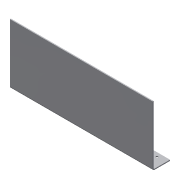
# Autodesk Inventor part: 17-0028-0024
Saved by Autodesk Inventor 2016 SP2 (Build 200236200, 236)
## iProperties
Category: IOP
Company: Universiteit van Amsterdam
Created: 2017-11-02
Part Number: 17-0028-0024
Material: Aluminum-6061-T6
Document SubType Name: Sheet Metal
Designer: Daan Giesen
Density: 2.71 g/cm^3
Sheet Metal Rule: Default_mm
Appearance: Aluminum - Flat - Version 1.1
Mass: 225.611 g
Surface Area: 873.904 cm^2
Volume: 83.2511 cm^3
Project: Digital PID Loop
Cost Center: 17-0028
User Status: Work in Progress
Authority: Reichsöllner, Lukas
Description: single bank frame
Author: Daan Giesen
Title: Digital PID Loop
Revision Number: A
Autodesk Inventor part; units mm, degrees
ref_plane "YZ Plane" through (0, 0, 0) normal (1, 0, 0) x (0, 1, 0)
ref_plane "XZ Plane" through (0, 0, 0) normal (0, 1, 0) x (-1, 0, 0)
ref_plane "XY Plane" through (0, 0, 0) normal (0, 0, 1) x (1, 0, 0)
sketch "Sketch1" plane through (0, 0, 0) normal (0, 0, 1) x (1, 0, 0)
  line L0 (0, 84) -> (0, -84) construction
  line L1 (-198.8, 0) -> (198.8, 0) construction
  line L2 (-142, -60) -> (142, -60)
  line L3 (142, -60) -> (142, 60)
  line L4 (142, 60) -> (-142, 60)
  line L5 (-142, 60) -> (-142, -60)
  line L6 (-142, -60) -> (142, 60) construction
  line L7 (142, -60) -> (-142, 60) construction
  point P0 (0, 0)
  dimension "d0" = 284
  dimension "d1" = 120
  measures "d0" distance of L3.end L4.end
  measures "d1" distance of L2.end L3.end
extrude "Plate1" add sketch "Sketch1" along normal blind 2
sketch "Sketch2" plane through (-142, -58, 2) normal (0, -1, 0) x (1, 0, 0)
  line L0 (284, 0) -> (0, 0)
  line L1 (0, 0) -> (0, -35)
  line L2 (0, -35) -> (284, -35)
  line L3 (284, -35) -> (284, 0)
  constraints: 6 end point, 1 horizontal, 1 perpendicular, 1 vertical
edge flange "Flange1" height 35 angle 90 thickness 2 bend radius 2 thickness toward (0, -1, 0) relief tear relief width 2 relief depth 1 edges at (0, -60, 0) wall of the first edge with corners at (142, -58, 2) (-142, -58, 2) (-142, -58, -33) (142, -58, -33)
bend "Bend1"
corner "Corner1"
sketch "Sketch5" plane through (0, 0, 2) normal (0, 0, 1) x (1, 0, 0)
  circle A0 centre (-111.95, 42.639) radius 2 projected
  circle A1 centre (-85.95, 42.639) radius 2 projected
  circle A2 centre (-59.95, 42.639) radius 2 projected
  circle A3 centre (-33.95, 42.639) radius 2 projected
  circle A4 centre (-7.95, 42.639) radius 2 projected
  circle A5 centre (25.35, 42.639) radius 2 projected
  circle A6 centre (51.35, 42.639) radius 2 projected
  circle A7 centre (77.35, 42.639) radius 2 projected
  circle A8 centre (103.35, 42.639) radius 2 projected
  circle A9 centre (129.35, 42.639) radius 2 projected
  circle A10 centre (116.35, 42.639) radius 2 projected
  circle A11 centre (90.35, 42.639) radius 2 projected
  circle A12 centre (64.35, 42.639) radius 2 projected
  circle A13 centre (38.35, 42.639) radius 2 projected
  circle A14 centre (12.35, 42.639) radius 2 projected
  circle A15 centre (-20.95, 42.639) radius 2 projected
  circle A16 centre (-46.95, 42.639) radius 2 projected
  circle A17 centre (-72.95, 42.639) radius 2 projected
  circle A18 centre (-98.95, 42.639) radius 2 projected
  circle A19 centre (-124.95, 42.639) radius 2 projected
  circle A20 centre (12, 52) radius 2.65 projected
  circle A21 centre (52, 52) radius 2.65 projected
  circle A22 centre (92, 52) radius 2.65 projected
  circle A23 centre (132, 52) radius 2.65 projected
  circle A24 centre (112, 26) radius 2.65 projected
  circle A25 centre (72, 26) radius 2.65 projected
  circle A26 centre (32, 26) radius 2.65 projected
  circle A27 centre (-8, 26) radius 2.65 projected
  circle A28 centre (-48, 26) radius 2.65 projected
  circle A29 centre (-28, 52) radius 2.65 projected
  circle A30 centre (-68, 52) radius 2.65 projected
  circle A31 centre (-88, 52) radius 2.65 projected
  circle A32 centre (-108, 52) radius 2.65 projected
  circle A33 centre (-128, 52) radius 2.65 projected
  circle A34 centre (-118, -8) radius 2.65 projected
  circle A35 centre (-95.7, 5) radius 2.65 projected
  circle A36 centre (-69.7, 5) radius 2.65 projected
  circle A37 centre (-43.7, 5) radius 2.65 projected
  circle A38 centre (-17.7, 5) radius 2.65 projected
  circle A39 centre (2.3, 5) radius 2.65 projected
  circle A40 centre (28.3, 5) radius 2.65 projected
  circle A41 centre (54.3, 5) radius 2.65 projected
  circle A42 centre (80.3, 5) radius 2.65 projected
  circle A43 centre (106.3, 5) radius 2.65 projected
  circle A44 centre (132.3, 5) radius 2.65 projected
  circle A45 centre (136, -8) radius 2.65 projected
  circle A46 centre (110, -8) radius 2.65 projected
  circle A47 centre (84, -8) radius 2.65 projected
  circle A48 centre (58, -8) radius 2.65 projected
  circle A49 centre (32, -8) radius 2.65 projected
  circle A50 centre (6, -8) radius 2.65 projected
  circle A51 centre (-14, -8) radius 2.65 projected
  circle A52 centre (-40, -8) radius 2.65 projected
  circle A53 centre (-66, -8) radius 2.65 projected
  circle A54 centre (-92, -8) radius 2.65 projected
  circle A55 centre (-121.7, 5) radius 2.65 projected
  circle A56 centre (-128, 26) radius 2.65 projected
  circle A57 centre (-108, 26) radius 2.65 projected
  circle A58 centre (-88, 26) radius 2.65 projected
  circle A59 centre (-48, 52) radius 2.65 projected
  circle A60 centre (-68, 26) radius 2.65 projected
  circle A61 centre (-28, 26) radius 2.65 projected
  circle A62 centre (12, 26) radius 2.65 projected
  circle A63 centre (52, 26) radius 2.65 projected
  circle A64 centre (92, 26) radius 2.65 projected
  circle A65 centre (132, 26) radius 2.65 projected
  circle A66 centre (112, 52) radius 2.65 projected
  circle A67 centre (72, 52) radius 2.65 projected
  circle A68 centre (32, 52) radius 2.65 projected
  circle A69 centre (-8, 52) radius 2.65 projected
  line L0 (-142, -15) -> (142, -15) projected
  line L1 (-142, 60) -> (-142, -15) projected
  line L2 (142, 60) -> (-142, 60) construction
  line L3 (142, -15) -> (142, 60) projected
  line L4 (142, -47.8) -> (142, -19.2) projected
  arc A70 (142, -19.2) -> (139.8, -17) centre (139.8012, -19.1988) ccw projected
  line L5 (139.8, -17) -> (-139.8, -17) construction
  arc A71 (-139.8, -17) -> (-142, -19.2) centre (-139.8012, -19.1988) ccw projected
  line L6 (-142, -19.2) -> (-142, -47.8) projected
  arc A72 (-142, -47.8) -> (-139.8, -50) centre (-139.8012, -47.8012) ccw projected
  line L7 (-139.8, -50) -> (139.8, -50) projected
  arc A73 (139.8, -50) -> (142, -47.8) centre (139.8012, -47.8012) ccw projected
  circle A74 centre (138, -46) radius 1.6 projected
  circle A75 centre (123.9, -21.55) radius 0.5 projected
  circle A76 centre (84.9, -21.55) radius 0.5 projected
  circle A77 centre (93.4, -21.55) radius 0.5 projected
  circle A78 centre (138, -21) radius 1.6 projected
  circle A79 centre (132.4, -21.55) radius 0.5 projected
  circle A80 centre (106.4, -21.55) radius 0.5 projected
  circle A81 centre (119.4, -21.55) radius 0.5 projected
  circle A82 centre (110.9, -21.55) radius 0.5 projected
  circle A83 centre (45.9, -21.55) radius 0.5 projected
  circle A84 centre (54.4, -21.55) radius 0.5 projected
  circle A85 centre (1, -46) radius 1.6 projected
  circle A86 centre (28.4, -21.55) radius 0.5 projected
  circle A87 centre (1, -27) radius 1.6 projected
  circle A88 centre (71.9, -21.55) radius 0.5 projected
  circle A89 centre (80.4, -21.55) radius 0.5 projected
  circle A90 centre (-13.4, -21.55) radius 0.5 projected
  circle A91 centre (19.9, -21.55) radius 0.5 projected
  circle A92 centre (-4.9, -21.55) radius 0.5 projected
  circle A93 centre (97.9, -21.55) radius 0.5 projected
  circle A94 centre (128.15, -21.55) radius 0.5 projected
  circle A95 centre (58.9, -21.55) radius 0.5 projected
  circle A96 centre (67.4, -21.55) radius 0.5 projected
  circle A97 centre (102.15, -21.55) radius 0.5 projected
  circle A98 centre (115.15, -21.55) radius 0.5 projected
  circle A99 centre (89.15, -21.55) radius 0.5 projected
  circle A100 centre (76.15, -21.55) radius 0.5 projected
  circle A101 centre (63.15, -21.55) radius 0.5 projected
  circle A102 centre (41.4, -21.55) radius 0.5 projected
  circle A103 centre (50.15, -21.55) radius 0.5 projected
  circle A104 centre (6.9, -21.55) radius 0.5 projected
  circle A105 centre (32.9, -21.55) radius 0.5 projected
  circle A106 centre (15.4, -21.55) radius 0.5 projected
  circle A107 centre (24.15, -21.55) radius 0.5 projected
  circle A108 centre (37.15, -21.55) radius 0.5 projected
  circle A109 centre (-9.15, -21.55) radius 0.5 projected
  circle A110 centre (11.15, -21.55) radius 0.5 projected
  circle A111 centre (1, -21) radius 0.5 projected
  circle A112 centre (-52.4, -21.55) radius 0.5 projected
  circle A113 centre (-43.9, -21.55) radius 0.5 projected
  circle A114 centre (-128, -46) radius 1.6 projected
  circle A115 centre (-69.9, -21.55) radius 0.5 projected
  circle A116 centre (-78.4, -21.55) radius 0.5 projected
  circle A117 centre (-65.4, -21.55) radius 0.5 projected
  circle A118 centre (-108.9, -21.55) radius 0.5 projected
  circle A119 centre (-117.4, -21.55) radius 0.5 projected
  circle A120 centre (-121.9, -21.55) radius 0.5 projected
  circle A121 centre (-134, -46.5) radius 0.6 projected
  circle A122 centre (-134, -43) radius 0.6 projected
  circle A123 centre (-134, -39.5) radius 0.6 projected
  circle A124 centre (-134.46, -30.54) radius 0.8 projected
  circle A125 centre (-138.5, -34) radius 0.5 projected
  circle A126 centre (-137, -28) radius 0.75 projected
  circle A127 centre (-134.46, -25.46) radius 0.8 projected
  circle A128 centre (-139.54, -30.54) radius 0.8 projected
  circle A129 centre (-138, -21) radius 1.6 projected
  circle A130 centre (-139.54, -25.46) radius 0.8 projected
  circle A131 centre (-30.9, -21.55) radius 0.5 projected
  circle A132 centre (-26.4, -21.55) radius 0.5 projected
  circle A133 centre (-56.9, -21.55) radius 0.5 projected
  circle A134 centre (-39.4, -21.55) radius 0.5 projected
  circle A135 centre (-17.9, -21.55) radius 0.5 projected
  circle A136 centre (-22.15, -21.55) radius 0.5 projected
  circle A137 centre (-48.15, -21.55) radius 0.5 projected
  circle A138 centre (-35.15, -21.55) radius 0.5 projected
  circle A139 centre (-61.15, -21.55) radius 0.5 projected
  circle A140 centre (-91.4, -21.55) radius 0.5 projected
  circle A141 centre (-82.9, -21.55) radius 0.5 projected
  circle A142 centre (-130.4, -21.55) radius 0.5 projected
  circle A143 centre (-95.9, -21.55) radius 0.5 projected
  circle A144 centre (-104.4, -21.55) radius 0.5 projected
  circle A145 centre (-74.15, -21.55) radius 0.5 projected
  circle A146 centre (-87.15, -21.55) radius 0.5 projected
  circle A147 centre (-113.15, -21.55) radius 0.5 projected
  circle A148 centre (-100.15, -21.55) radius 0.5 projected
  circle A149 centre (-126.15, -21.55) radius 0.5 projected
  point P0 (0, 0)
extrude "Cut1" cut sketch "Sketch5" against normal blind 2 contours A0 | A1 | A2 | A3 | A4 | A5 | A6 | A7 | A8 | A9 | A10 | A11 | A12 | A13 | A14 | A15 | A16 | A17 | A18 | A19 | A20 | A21 | A22 | A23 | A24 | A25 | A26 | A27 | A28 | A29 | A30 | A31 | A32 | A33 | A34 | A35 | A36 | A37 | A38 | A39 | A40 | A41 | A42 | A43 | A44 | A45 | A46 | A47 | A48 | A49 | A50 | A51 | A52 | A53 | A54 | A55 | A56 | A57 | A58 | A59 | A60 | A61 | A62 | A63 | A64 | A65 | A66 | A67 | A68 | A69 | A74 | A78 | A85 | A87 | A114 | A129
sketch "Sketch6" plane through (-142, -58, -33) normal (0, 1, 0) x (1, 0, 0)
  line L0 (284, 0) -> (0, 0) projected
  line L1 (0, 0) -> (0, -31) projected
  point P0 (142, -33)
  point P1 (18, -8)
  point P2 (88, -8)
  dimension "d17" = 8
  dimension "d18" = 18
  dimension "d26" = 70
  constraints: 1 horizontal alignment
  measures "d17" distance from line of L0 point (18, -8)
  measures "d18" distance from line of L1 point (18, -8)
  measures "d26" distance of point (18, -8) point (88, -8)
hole "Hole1" at (-124, -58, -25) at (-54, -58, -25) direction (0, -1, 0) diameter 4.3 end through all
mirror "Mirror1" about plane through (0, 0, 0) normal (1, 0, 0) of "Hole1"
equation "\"d15\" = Thickness"
equation "\"d24\" = Thickness"
equation "\"d3\" = BendReliefWidth"
equation "\"d4\" = BendReliefDepth"
equation "\"d5\" = MinimumRemnant"
equation "\"d6\" = BendRadius"
equation "\"d9\" = BendRadius"
equation "\"d10\" = CornerReliefSize"
equation "\"d11\" = GapSize"
equation "\"d12\" = JacobiRadiusSize"
equation "\"BendRadius\" = Thickness"
equation "\"BendReliefWidth\" = Thickness"
equation "\"BendReliefDepth\" = 0.5 * Thickness"
equation "\"CornerReliefSize\" = 4 * Thickness"
equation "\"MinimumRemnant\" = 2 * Thickness"
equation "\"TransitionRadius\" = BendRadius"
equation "\"JacobiRadiusSize\" = BendRadius"
equation "\"GapSize\" = Thickness"
equation "\"d2\" = BendRadius"
equation "\"Thickness\" = 2"
body "Solid1"
